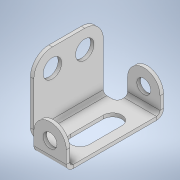
# Autodesk Inventor part: 26886-Vodička_Vojtěch_příklad-3
Saved by Autodesk Inventor 2022 (Build 260153000, 153)
## iProperties
Created: 2022-03-24
Part Number: 26886-Vodička_Vojtěch_příklad-3
Material: Všeobecné
Document SubType Name: Sheet Metal
Designer: vojta
Density: 1 g/cm^3
Sheet Metal Rule: Výchozí_mm
Appearance: Výchozí
Author: vojta
Autodesk Inventor part; units mm, degrees
ref_plane "YZ Plane" through (0, 0, 0) normal (1, 0, 0) x (0, 1, 0)
ref_plane "XZ Plane" through (0, 0, 0) normal (0, 1, 0) x (-1, 0, 0)
ref_plane "XY Plane" through (0, 0, 0) normal (0, 0, 1) x (1, 0, 0)
sketch "Náčrt1" plane through (0, 0, 0) normal (0, 1, 0) x (-1, 0, 0)
  line L0 (0, 0) -> (28, 0)
  line L1 (43, -12) -> (43, -72)
  line L2 (28, -84) -> (0, -84)
  line L3 (0, -84) -> (0, 0)
  line L4 (43, -12) -> (32, -12)
  line L5 (28, -8) -> (28, 0)
  line L6 (28, -84) -> (28, -76)
  line L7 (32, -72) -> (43, -72)
  arc A0 (24, -28) -> (8, -28) centre (16, -28) ccw
  arc A1 (8, -56) -> (24, -56) centre (16, -56) ccw
  line L8 (24, -28) -> (24, -56)
  line L9 (8, -28) -> (8, -56)
  arc A2 (28, -8) -> (32, -12) centre (32, -8) ccw
  arc A3 (32, -72) -> (28, -76) centre (32, -76) ccw
  point P0 (28, -12)
  point P1 (28, -72)
  dimension "d3" = 15
  dimension "d4" = 12
  dimension "d5" = 84
  dimension "d6" = 43
  dimension "d7" = 60
  dimension "d10" = 16
  dimension "d11" = 16
  dimension "d12" = 28
  dimension "d13" = 16
  dimension "d15" = 4
  measures "d3" distance of L1.start point (28, -12)
  measures "d4" distance of L2.start point (28, -72)
  measures "d5" distance between parallel lines of L2 L0
  measures "d6" distance between parallel lines of L3 L1
  measures "d7" distance between parallel lines of L7 L4
  measures "d10" diameter of A0
  measures "d11" diameter of A1
  measures "d12" distance of A1.centre A0.centre
  measures "d13" distance from line of L3 A0.centre
  measures "d15" radius of A2
extrude "Deska1" add sketch "Náčrt1" along normal blind 3
sketch "Náčrt2" plane through (0, 0, -3) normal (0, 0, 1) x (1, 0, 0)
  line L0 (-28, 0) -> (0, 0)
  line L1 (0, 0) -> (0, 31)
  line L2 (0, 31) -> (-28, 31)
  line L3 (-28, 31) -> (-28, 0)
  constraints: 6 end point, 1 horizontal, 1 perpendicular, 1 vertical
edge flange "Obruba1" height 31 angle 90 thickness 3 bend radius 3 thickness toward (0, 0, 1) relief tear relief width 3 relief depth 1.5 corner gap 3 corner form 0 edges at (-14, 3, 0) (-14, 3, -84) wall of the first edge with corners at (-28, 0, -3) (0, 0, -3) (0, 31, -3) (-28, 31, -3)
bend "Ohyb1"
corner "Roh1"
fillet "Zaoblení rohu1" radius 14 4 edges at (-28, 31, -1.5) (0, 31, -1.5) (-28, 31, -82.5) (0, 31, -82.5)
sketch "Náčrt3" plane through (0, 6, -84) normal (0, 0, -1) x (-1, 0, 0)
  line L0 (28, -6) -> (0, -6) projected
  line L1 (28, 11) -> (28, 0) projected
  point P0 (14, 11)
  dimension "d27" = 17
  dimension "d28" = 14
  measures "d27" distance from line of L0 point (14, 11)
  measures "d28" distance from line of L1 point (14, 11)
hole "Díra1" at (-14, 17, -84) direction (0, 0, 1) diameter 12 depth 3 tip angle 118
sketch "Náčrt4" plane through (-28, 6, 0) normal (0, 0, 1) x (1, 0, 0)
  line L0 (28, -6) -> (0, -6) projected
  line L1 (28, 11) -> (28, 0) projected
  point P0 (14, 11)
  dimension "d36" = 17
  dimension "d37" = 14
  measures "d36" distance from line of L0 point (14, 11)
  measures "d37" distance from line of L1 point (14, 11)
hole "Díra2" at (-14, 17, 0) direction (0, 0, -1) diameter 12 depth 3 tip angle 118
sketch "Náčrt5" plane through (-40, 0, -12) normal (-1, 0, 0) x (0, -1, 0)
  line L0 (0, -60) -> (0, 0)
  line L1 (0, 0) -> (-60, 0)
  line L2 (-60, 0) -> (-60, -60)
  line L3 (-60, -60) -> (0, -60)
  constraints: 6 end point, 1 horizontal, 1 perpendicular, 1 vertical
edge flange "Obruba2" height 60 angle 90 thickness 3 bend radius 3 thickness toward (-1, 0, 0) relief tear relief width 3 relief depth 1.5 edges at (-43, 3, -42) wall of the first edge with corners at (-40, 0, -72) (-40, 0, -12) (-40, 60, -12) (-40, 60, -72)
bend "Ohyb2"
corner "Roh2"
fillet "Zaoblení rohu2" radius 16 2 edges at (-41.5, 60, -72) (-41.5, 60, -12)
sketch "Náčrt6" plane through (-43, 6, -72) normal (-1, 0, 0) x (0, 0, 1)
  line L0 (60, -6) -> (0, -6) projected
  line L1 (0, 0) -> (0, 38) projected
  point P0 (72, -6)
  point P1 (16, 38)
  dimension "d56" = 44
  dimension "d57" = 16
  measures "d56" distance from line of L0 point (16, 38)
  measures "d57" distance from line of L1 point (16, 38)
hole "Díra3" at (-43, 44, -56) direction (1, 0, 0) diameter 16 depth 3 tip angle 118
sketch "Náčrt7" plane through (-43, 6, -72) normal (-1, 0, 0) x (0, 0, 1)
  line L0 (60, -6) -> (0, -6) projected
  line L1 (60, 38) -> (60, 0) projected
  point P0 (72, -6)
  point P1 (44, 38)
  dimension "d65" = 44
  dimension "d66" = 16
  measures "d65" distance from line of L0 point (44, 38)
  measures "d66" distance from line of L1 point (44, 38)
hole "Díra4" at (-43, 44, -28) direction (1, 0, 0) diameter 16 depth 3 tip angle 118
equation "\"d34\" = Tloušťka"
equation "\"d43\" = Tloušťka"
equation "\"d63\" = Tloušťka"
equation "\"d72\" = Tloušťka"
equation "\"d14\" = Tloušťka"
equation "\"d16\" = ŠířkaVýštipu"
equation "\"d17\" = HloubkaVýštipu"
equation "\"d18\" = MinimálníZbytek"
equation "\"d19\" = PřechodovýPoloměr"
equation "\"d22\" = PoloměrOhybu"
equation "\"d23\" = VelikostRohovéhoVýštipu"
equation "\"d24\" = VelikostMezery"
equation "\"d25\" = VelikostJacobihoPoloměru"
equation "\"d45\" = ŠířkaVýštipu"
equation "\"d46\" = HloubkaVýštipu"
equation "\"d47\" = MinimálníZbytek"
equation "\"d48\" = PřechodovýPoloměr"
equation "\"d51\" = PoloměrOhybu"
equation "\"d52\" = VelikostRohovéhoVýštipu"
equation "\"d53\" = VelikostMezery"
equation "\"d54\" = VelikostJacobihoPoloměru"
equation "\"PoloměrOhybu\" = Tloušťka"
equation "\"ŠířkaVýštipu\" = Tloušťka"
equation "\"HloubkaVýštipu\" = 0.5 * Tloušťka"
equation "\"VelikostRohovéhoVýštipu\" = 4 * Tloušťka"
equation "\"MinimálníZbytek\" = 2 * Tloušťka"
equation "\"PřechodovýPoloměr\" = PoloměrOhybu"
equation "\"VelikostJacobihoPoloměru\" = PoloměrOhybu"
equation "\"VelikostMezery\" = Tloušťka"
equation "\"Tloušťka\" = 3"
